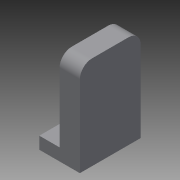
# Autodesk Inventor part: 130
Saved by Autodesk Inventor 2014 (Build 180170000, 170)
## iProperties
Created: 2017-04-22
Part Number: 130
Material: Generic
Document SubType Name: Modeling
Designer: Andy
Density: 1 g/cm^3
Appearance: Default
Author: Andy
Autodesk Inventor part; units mm, degrees
ref_plane "YZ Plane" through (0, 0, 0) normal (1, 0, 0) x (0, 1, 0)
ref_plane "XZ Plane" through (0, 0, 0) normal (0, 1, 0) x (-1, 0, 0)
ref_plane "XY Plane" through (0, 0, 0) normal (0, 0, 1) x (1, 0, 0)
sketch "Sketch1" plane through (0, 0, 0) normal (1, 0, 0) x (0, 1, 0)
  line L0 (0, 10) -> (0, 0)
  line L1 (0, 0) -> (7.5, 0)
  line L2 (7.5, 0) -> (7.5, 10)
  arc A0 (1.5, 11.5) -> (0, 10) centre (1.5, 10) ccw
  line L3 (1.5, 10) -> (1.5, 11.5) construction
  line L4 (1.5, 10) -> (0, 10) construction
  arc A1 (7.5, 10) -> (6, 11.5) centre (6, 10) ccw
  line L5 (6, 10) -> (6, 11.5) construction
  line L6 (6, 10) -> (7.5, 10) construction
  line L7 (1.5, 11.5) -> (6, 11.5)
  dimension "d0" = 7.5
  dimension "d1" = 90
  dimension "d2" = 90
  constraints: 16 end point, 4 point on circle, 2 centre point, 2 tangent, 1 parallel, 1 perpendicular, 1 vertical
  measures "d0" distance of L0.end L1.end
  measures "d1" angle of L3 L4
  measures "d2" angle of L6 L5
extrude "Extrusion1" add sketch "Sketch1" along normal blind 5
sketch "Sketch2" plane through (0, 0, 0) normal (-1, 0, 0) x (0, 0, 1)
  line L0 (10, 7.5) -> (0, 7.5) projected
  line L1 (1.5, 7.5) -> (11.5, 7.5)
  line L2 (11.5, 7.5) -> (11.5, 0)
  line L3 (11.5, 0) -> (1.5, 0)
  line L4 (1.5, 0) -> (1.5, 7.5)
  constraints: 8 end point, 2 parallel, 1 horizontal, 1 perpendicular, 1 point on line
extrude "Extrusion2" cut sketch "Sketch2" against normal blind 2.5
body "Solid1"
